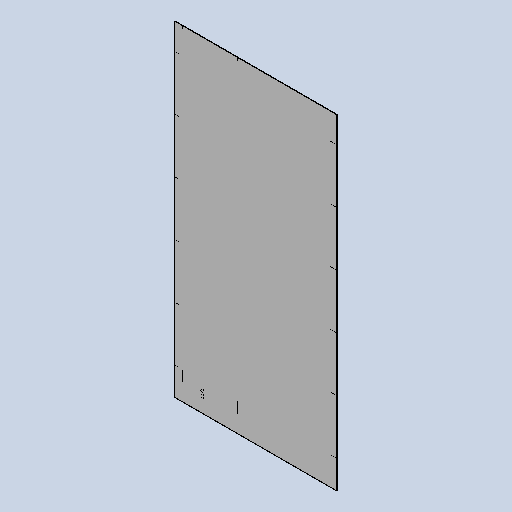
# Autodesk Inventor part: GBK 2122 shield 2
Saved by Autodesk Inventor 2026.2 (Build 302298010, 298A)
## iProperties
Manager: 4
Created: 2026-04-17
Part Number: GBK 2122 shield 2
Material: Steel
Document SubType Name: Sheet Metal
Designer: pokla
Stock Number: 2122
Mass: 138487 g
Surface Area: 88564.8 cm^2
Volume: 17641.6 cm^3
Density: 7.85 g/cm^3
Sheet Metal Rule: Default_mm
Sheet Metal Width: 1480,000 mm
Sheet Metal Length: 2980,000 mm
Sheet Metal Area: 4410400,000 mm^2
Appearance: Default
Flat Pattern Width: 148 cm
Flat Pattern Length: 298 cm
Flat Pattern Area: 44104 cm^2
Project: 3
Author: admin
Autodesk Inventor part; units mm, degrees
ref_plane "YZ Plane" through (0, 0, 0) normal (1, 0, 0) x (0, 1, 0)
ref_plane "XZ Plane" through (0, 0, 0) normal (0, 1, 0) x (-1, 0, 0)
ref_plane "XY Plane" through (0, 0, 0) normal (0, 0, 1) x (1, 0, 0)
sketch "Sketch1" plane through (0, 0, 0) normal (0, 0, 1) x (1, 0, 0)
  line L0 (740, -1490) -> (-740, -1490)
  line L1 (-740, -1490) -> (-740, 1490)
  line L2 (-740, 1490) -> (740, 1490)
  line L3 (740, 1490) -> (740, -1490)
  line L4 (740, -1490) -> (-740, 1490) construction
  line L5 (-740, -1490) -> (740, 1490) construction
  point P0 (0, 0)
  dimension "d0" = 1480
  dimension "d1" = 2980
  measures "d0" distance of L1.end L2.end
  measures "d1" distance of L0.end L1.end
extrude "Plate1" add sketch "Sketch1" along normal blind 4
sketch "Sketch2" plane through (0, 0, 0) normal (0, 0, -1) x (-1, 0, 0)
  line L0 (512.6266, -1291.8213) -> (512.6266, -1649.5118) construction
  line L1 (512.6266, -1649.5118) -> (521.7001, -1649.5118) construction
  line L2 (521.7001, -1649.5118) -> (521.7001, -1291.8213) construction
  line L3 (521.7001, -1291.8213) -> (512.6266, -1291.8213) construction
  point P0 (0, 0)
  constraints: 2 other
mark "Mark1"
sketch "Эскиз3" plane through (0, 0, 0) normal (0, 0, -1) x (-1, 0, 0)
  line L0 (710, -1234.5) -> (770, -1234.5) projected
  line L1 (710, -1234.5) -> (710, -1230.5) projected
  line L2 (710, -737.8333) -> (770, -737.8333) projected
  line L3 (710, -737.8333) -> (710, -733.8333) projected
  line L4 (710, -241.1667) -> (770, -241.1667) projected
  line L5 (710, -241.1667) -> (710, -237.1667) projected
  line L6 (710, 255.5) -> (770, 255.5) projected
  line L7 (710, 255.5) -> (710, 259.5) projected
  line L8 (710, 752.1667) -> (770, 752.1667) projected
  line L9 (710, 752.1667) -> (710, 756.1667) projected
  line L10 (710, 1248.8333) -> (770, 1248.8333) projected
  line L11 (710, 1248.8333) -> (710, 1252.8333) projected
  line L12 (669.8628, -1238) -> (669.8628, -1335) projected
  line L13 (669.8628, -1335) -> (665.8638, -1335) projected
  line L14 (169.7342, -1238) -> (169.7342, -1335) projected
  line L15 (169.7342, -1335) -> (165.7352, -1335) projected
  line L16 (-330.3944, -1238) -> (-330.3944, -1335) projected
  line L17 (-330.3944, -1335) -> (-334.3934, -1335) projected
  ellipse E0 centre (669.8628, 1490.5) end of major axis (669.8628, 1520.5) minor radius 0.6803 (669.8628, 1460.5) -> (669.8628, 1520.5) ccw projected
  line L18 (669.8628, 1460.5) -> (665.8638, 1460.5) projected
  line L19 (-738.6395, 1248.8333) -> (-680, 1248.8333) projected
  line L20 (-680, 1248.8333) -> (-680, 1252.8333) projected
  line L21 (-738.6395, 752.1667) -> (-680, 752.1667) projected
  line L22 (-680, 752.1667) -> (-680, 756.1667) projected
  line L23 (-738.6395, 255.5) -> (-680, 255.5) projected
  line L24 (-680, 255.5) -> (-680, 259.5) projected
  line L25 (-738.6395, -241.1667) -> (-680, -241.1667) projected
  line L26 (-680, -241.1667) -> (-680, -237.1667) projected
  line L27 (-738.6395, -737.8333) -> (-680, -737.8333) projected
  line L28 (-680, -737.8333) -> (-680, -733.8333) projected
  line L29 (-738.6395, -1234.5) -> (-680, -1234.5) projected
  line L30 (-680, -1234.5) -> (-680, -1230.5) projected
  ellipse E1 centre (169.7342, 1490.5) end of major axis (169.7342, 1520.5) minor radius 0.6803 (169.7342, 1460.5) -> (169.7342, 1520.5) ccw projected
  line L31 (169.7342, 1460.5) -> (165.7352, 1460.5) projected
  ellipse E2 centre (-330.3944, 1490.5) end of major axis (-330.3944, 1520.5) minor radius 0.6803 (-330.3944, 1460.5) -> (-330.3944, 1520.5) ccw projected
  line L32 (-330.3944, 1460.5) -> (-334.3934, 1460.5) projected
  point P0 (0, 0)
  constraints: 3 other
mark "Маркировка2"
equation "\"d0\" = Лист_ширина"
equation "\"d2\" = Thickness"
equation "\"BendRadius\" = Thickness"
equation "\"BendReliefWidth\" = Thickness"
equation "\"BendReliefDepth\" = 0.5 * Thickness"
equation "\"CornerReliefSize\" = 4 * Thickness"
equation "\"MinimumRemnant\" = 2 * Thickness"
equation "\"TransitionRadius\" = BendRadius"
equation "\"JacobiRadiusSize\" = BendRadius"
equation "\"GapSize\" = Thickness"
equation "\"Лист_ширина\" = 1480"
equation "\"Thickness\" = 4"
body "Solid1"
